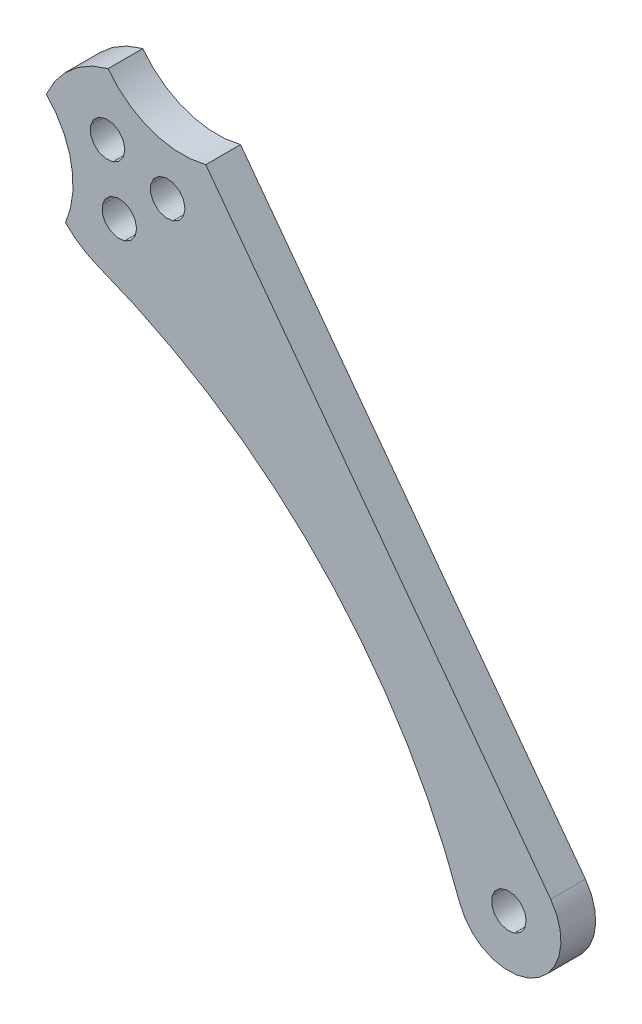
# Autodesk Inventor part: Part4
Saved by Autodesk Inventor 2020 (Build 240168000, 168)
## iProperties
Created: 2020-01-24
Part Number: Part4
Material: 一般
Document SubType Name: Modeling
Designer: tanjihayato
Density: 1 g/cm^3
Appearance: 既定
Author: tanjihayato
Autodesk Inventor part; units mm, degrees
ref_plane "YZ Plane" through (0, 0, 0) normal (1, 0, 0) x (0, 1, 0)
ref_plane "XZ Plane" through (0, 0, 0) normal (0, 1, 0) x (-1, 0, 0)
ref_plane "XY Plane" through (0, 0, 0) normal (0, 0, 1) x (1, 0, 0)
sketch "スケッチ1" plane through (0, 0, 0) normal (0, 0, 1) x (1, 0, 0)
  circle A0 centre (-11.4931, -19.1593) radius 14 construction
  circle A1 centre (16.245, -15.3385) radius 14 construction
  line L0 (-197.2268, -33.1593) -> (179.6604, -33.1593) construction
  line L1 (-67.2952, 44.8622) -> (-67.2952, -57.3934) construction
  circle A2 centre (-59.2702, 32.0272) radius 2 construction
  circle A3 centre (-59.2702, 32.0272) radius 5.025 construction
  line L2 (-77.2952, 24.5844) -> (-77.2952, -15.0909)
  circle A4 centre (-59.2702, 32.0272) radius 4 construction
  circle A5 centre (-28.0204, 0.0121) radius 22.342 construction
  circle A6 centre (-40.2768, 3.1689) radius 22.342 construction
  circle A7 centre (-60.3241, 13.0314) radius 14 construction
  circle A8 centre (-53.8442, -14.5819) radius 14 construction
  circle A9 centre (-39.4931, -19.1593) radius 14 construction
  circle A10 centre (-62.0279, -1.9354) radius 14 construction
  line L3 (-50.4137, 33.1763) -> (-63.8556, 5.853) construction
  line L4 (-63.8556, 5.853) -> (-60.2002, -9.7238) construction
  line L5 (-60.2002, -9.7238) -> (-47.4881, -19.44) construction
  line L6 (-47.4881, -19.44) -> (-24.0934, -18.6188) construction
  circle A11 centre (-60.3241, 13.0314) radius 8 construction
  circle A12 centre (-62.0279, -1.9354) radius 8 construction
  circle A13 centre (-53.8442, -14.5819) radius 8 construction
  circle A14 centre (-39.4931, -19.1593) radius 8 construction
  circle A15 centre (-47.4881, -19.44) radius 1.3
  circle A16 centre (-31.498, -18.8787) radius 1.3
  circle A17 centre (-60.2002, -9.7238) radius 1.3
  circle A18 centre (-63.8556, 5.853) radius 1.3
  circle A19 centre (-56.7927, 20.2097) radius 1.3
  circle A20 centre (-60.3241, 13.0314) radius 5
  circle A21 centre (-62.0279, -1.9354) radius 5
  circle A22 centre (-53.8442, -14.5819) radius 5
  circle A23 centre (-39.4931, -19.1593) radius 5
  circle A24 centre (-40.2768, 3.1689) radius 5.05
  circle A25 centre (-6.7239, 1.3907) radius 28.55 construction
  circle A26 centre (32.5545, 13.5882) radius 32.1 construction
  line L7 (-170.915, -81.4118) -> (490.0044, -81.4118) construction
  circle A27 centre (-1.9226, 44.1165) radius 2 construction
  circle A28 centre (71.1898, -32.1215) radius 2 construction
  circle A29 centre (45.6606, 13.5882) radius 1.5 construction
  circle A30 centre (22.3463, 32.4678) radius 2 construction
  line L8 (32.5545, 13.5882) -> (9.2401, 32.4678) construction
  line L9 (9.2401, 32.4678) -> (-15.0287, 44.1165) construction
  line L10 (32.5545, 13.5882) -> (58.0836, -32.1215) construction
  line L11 (-1.9226, 44.1165) -> (22.3463, 32.4678) construction
  line L12 (22.3463, 32.4678) -> (45.6606, 13.5882) construction
  line L13 (45.6606, 13.5882) -> (71.1898, -32.1215) construction
  circle A31 centre (-15.0287, 44.1165) radius 2
  circle A32 centre (9.2401, 32.4678) radius 2
  circle A33 centre (32.5545, 13.5882) radius 4.025
  circle A34 centre (58.0836, -32.1215) radius 2
  circle A35 centre (-15.0287, 44.1165) radius 4
  circle A36 centre (58.0836, -32.1215) radius 4
  arc A37 (-10.4642, 49.4236) -> (-16.7225, 50.9085) centre (-15.0287, 44.1165) ccw
  arc A38 (55.6895, -38.6994) -> (63.1356, -27.2762) centre (58.0836, -32.1215) ccw
  arc A39 (75.6915, -11.451) -> (23.3358, 45.6882) centre (45.6606, 13.5882) ccw construction
  arc A40 (5.9468, 46.5813) -> (23.3358, 45.6882) centre (15.2178, 57.3607) ccw construction
  line L14 (2.6419, 49.4236) -> (5.9468, 46.5813) construction
  arc A41 (2.6419, 49.4236) -> (-4.7411, 50.524) centre (-1.9226, 44.1165) ccw construction
  arc A42 (75.6915, -11.451) -> (76.2418, -27.2762) centre (84.8125, -19.056) ccw construction
  arc A43 (69.4805, -38.9096) -> (76.2418, -27.2762) centre (71.1898, -32.1215) ccw construction
  arc A44 (62.5853, -11.451) -> (8.8225, 44.6623) centre (32.5545, 13.5882) ccw
  arc A45 (-7.1594, 46.5813) -> (10.2296, 45.6882) centre (2.1116, 57.3607) ccw construction
  line L15 (-7.1594, 46.5813) -> (-10.4642, 49.4236)
  arc A46 (62.5853, -11.451) -> (63.1356, -27.2762) centre (71.7064, -19.056) ccw
  arc A47 (-61.212, 39.8137) -> (-64.6423, 37.9887) centre (-59.2702, 32.0272) ccw
  circle A48 centre (-72.7952, 24.5844) radius 1.5
  arc A49 (-75.8076, 27.9274) -> (-77.2952, 24.5844) centre (-72.7952, 24.5844) ccw
  line L16 (-16.7225, 50.9085) -> (-61.212, 39.8137)
  circle A50 centre (-72.7952, 24.5844) radius 3 construction
  arc A51 (-77.2952, -15.0909) -> (-76.0696, -18.1776) centre (-72.7952, -15.0909) ccw
  circle A52 centre (-72.7952, -15.0909) radius 1.5
  circle A53 centre (-72.7952, -15.0909) radius 3 construction
  line L17 (-64.6423, 37.9887) -> (-75.8076, 27.9274)
  line L18 (-60.6517, -33.1593) -> (40.4684, -33.1593)
  line L19 (40.4684, -33.1593) -> (55.6895, -38.6994)
  circle A54 centre (-6.7239, 1.3907) radius 7.5
  line L20 (-76.0696, -18.1776) -> (-62.8347, -32.2172)
  arc A55 (-62.8347, -32.2172) -> (-60.6517, -33.1593) centre (-60.6517, -30.1593) ccw
  circle A56 centre (-60.6517, -30.1593) radius 1.5
  circle A57 centre (-6.7239, 1.3907) radius 29.55 construction
  line L21 (-90.7052, -28.1593) -> (49.3281, -28.1593) construction
  circle A58 centre (-26.5251, 43.8261) radius 4.5 construction
  circle A59 centre (-26.5251, 43.8261) radius 1.5
  circle A60 centre (-7.4902, 35.432) radius 1.5
  circle A61 centre (-7.4902, 35.432) radius 4.5 construction
  circle A62 centre (9.2401, 32.4678) radius 4
  circle A63 centre (32.5545, 13.5882) radius 34.1 construction
  circle A64 centre (17.9034, -22.1232) radius 1.5
  circle A65 centre (17.9034, -22.1232) radius 4.5 construction
  circle A66 centre (46.6805, -30.6316) radius 1.5
  circle A67 centre (46.6805, -30.6316) radius 4.5 construction
  circle A68 centre (-25.2792, -27.1593) radius 1.5
  circle A69 centre (-25.2792, -27.1593) radius 4.5 construction
  circle A70 centre (-48.4615, 38.3556) radius 1.5
  circle A71 centre (-48.4615, 38.3556) radius 4.5 construction
  circle A72 centre (-59.2702, 32.0272) radius 4.2
  circle A73 centre (-6.7239, 1.3907) radius 8.7
  circle A74 centre (-40.2768, 3.1689) radius 6.05
  circle A75 centre (-25.2792, -27.1593) radius 3 construction
  circle A76 centre (-0.0212, 51.52) radius 8
  line L22 (32.5545, 13.5882) -> (-0.0212, 51.52) construction
  line L23 (-2.09, 53.929) -> (3.0995, 52.1072) construction
  line L24 (3.0995, 52.1072) -> (-1.073, 48.5239) construction
  line L25 (-1.073, 48.5239) -> (-2.09, 53.929) construction
  circle A77 centre (-2.09, 53.929) radius 1.5
  circle A78 centre (3.0995, 52.1072) radius 1.5
  circle A79 centre (-1.073, 48.5239) radius 1.5
  circle A80 centre (32.5545, 13.5882) radius 1.5
  circle A81 centre (32.5545, 13.5882) radius 4.5
  line L26 (6.3979, 56.2945) -> (36.1652, 16.2738)
  arc A82 (28.3135, 12.0835) -> (-2.8797, 44.0481) centre (-21.9277, -5.7426) ccw
  circle A83 centre (-2.09, 53.929) radius 4 construction
  circle A84 centre (3.0995, 52.1072) radius 4 construction
  circle A85 centre (-1.073, 48.5239) radius 4 construction
  arc A86 (-2.042, 59.2606) -> (6.3947, 56.2988) centre (4.3738, 64.0393) ccw
  arc A87 (-5.7143, 45.8997) -> (-7.3677, 54.687) centre (-13.0607, 49.0666) ccw
  point P0 (0, 0)
  point P1 (0, 0)
  dimension "d7" = 16
  dimension "d8" = 16
  dimension "d10" = 16
  dimension "d0" = 10.05
  dimension "d1" = 10
  dimension "d2" = 8
  dimension "d3" = 28
  dimension "d4" = 28
  dimension "d5" = 28
  dimension "d6" = 28
  dimension "d9" = 16
  dimension "d11" = 2.6
  dimension "d12" = 2.6
  dimension "d13" = 2.6
  dimension "d14" = 2.6
  dimension "d15" = 2.6
  dimension "d16" = 10
  dimension "d17" = 10
  dimension "d18" = 10
  dimension "d19" = 10
  dimension "d20" = 10.1
  dimension "d21" = 57.1
  dimension "d22" = 41.1287
  dimension "d23" = 64.2
  dimension "d24" = 95
  dimension "d25" = 4
  dimension "d26" = 4
  dimension "d27" = 8.05
  dimension "d28" = 4
  dimension "d29" = 8
  dimension "d30" = 8
  dimension "d31" = 3
  dimension "d32" = 3
  dimension "d33" = 3
  dimension "d34" = 3
  dimension "d35" = 3
  dimension "d36" = 6
  dimension "d37" = 9
  dimension "d38" = 3
  dimension "d39" = 6
  dimension "d40" = 15
  dimension "d41" = 6
  dimension "d42" = 3
  dimension "d43" = 1
  dimension "d44" = 5
  dimension "d45" = 9
  dimension "d46" = 3
  dimension "d47" = 3
  dimension "d48" = 9
  dimension "d49" = 8
  dimension "d50" = 2
  dimension "d51" = 3
  dimension "d52" = 9
  dimension "d53" = 3
  dimension "d54" = 9
  dimension "d55" = 3
  dimension "d56" = 9
  dimension "d57" = 3
  dimension "d58" = 9
  dimension "d59" = 160
  dimension "d60" = 8.4
  dimension "d61" = 1.2
  dimension "d62" = 1
  dimension "d63" = 6
  dimension "d64" = 6
  dimension "d65" = 16
  dimension "d66" = 50
  constraints: 85 centre point, 54 end point, 50 point on circle, 48 tangent, 40 coincident, 7 parallel, 6 point on line, 4 equal radius, 2 midpoint, 1 horizontal, 1 perpendicular, 1 vertical, 16 other
  measures "d0" diameter of A3
  measures "d1" distance between parallel lines of L2 L1
  measures "d2" diameter of A4
  measures "d3" diameter of A7
  measures "d4" diameter of A8
  measures "d5" diameter of A9
  measures "d6" diameter of A10
  measures "d9" diameter of A13
  measures "d11" diameter of A15
  measures "d12" diameter of A16
  measures "d13" diameter of A17
  measures "d14" diameter of A18
  measures "d15" diameter of A19
  measures "d16" diameter of A20
  measures "d17" diameter of A21
  measures "d18" diameter of A22
  measures "d19" diameter of A23
  measures "d20" diameter of A24
  measures "d21" diameter of A25
  measures "d22" distance of A25.centre L8.start
  measures "d23" diameter of A26
  measures "d24" distance from line of L7 L8.start
  measures "d25" diameter of A31
  measures "d26" diameter of A32
  measures "d27" diameter of A33
  measures "d28" diameter of A34
  measures "d29" diameter of A35
  measures "d30" diameter of A36
  measures "d31" radial gap between concentric circles of A35 A37
  measures "d32" radial gap between concentric circles of A36 A38
  measures "d33" radial gap between concentric circles of A3 A47
  measures "d34" diameter of A48
  measures "d35" radial gap between concentric circles of A48 A49
  measures "d36" diameter of A50
  measures "d37" diameter of A51
  measures "d38" diameter of A52
  measures "d39" diameter of A53
  measures "d40" diameter of A54
  measures "d41" diameter of A55
  measures "d42" diameter of A56
  measures "d43" radial gap between concentric circles of A25 A57
  measures "d44" distance between parallel lines of L0 L21
  measures "d45" diameter of A58
  measures "d46" diameter of A59
  measures "d47" diameter of A60
  measures "d48" diameter of A61
  measures "d49" diameter of A62
  measures "d50" radial gap between concentric circles of A26 A63
  measures "d51" diameter of A64
  measures "d52" diameter of A65
  measures "d53" diameter of A66
  measures "d54" diameter of A67
  measures "d55" diameter of A68
  measures "d56" diameter of A69
  measures "d57" diameter of A70
  measures "d58" diameter of A71
  measures "d59" angle of L18 L19
  measures "d60" diameter of A72
  measures "d61" radial gap between concentric circles of A54 A73
  measures "d62" radial gap between concentric circles of A24 A74
  measures "d63" diameter of A75
  measures "d64" distance from line of A75.centre L18
  measures "d65" diameter of A76
  measures "d66" distance of L22.start L22.end
extrude "押し出し1" add sketch "スケッチ1" along normal blind 3 contours A33 | A82 A76 L26 A81 | A81 | A76 A87 A86
